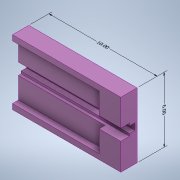
# Autodesk Inventor part: pistonHousing-8-in
Saved by Autodesk Inventor 2020.2 (Build 242310000, 310)
## iProperties
Created: 2020-01-13
Part Number: pistonHousing-8-in
Material: PET Plastic
Document SubType Name: Modeling
Designer: robst
Density: 1.541 g/cm^3
Appearance: Smooth - Purple
Author: robst
Autodesk Inventor part; units mm, degrees
ref_plane "Work Plane1" through (-127, 50.8, 9.525) normal (0, 0, 1) x (1, 0, 0)
sketch "Sketch1" plane through (0, 0, 0) normal (0, 0, 1) x (1, 0, 0)
  line L0 (-127, -76.2) -> (127, -76.2)
  line L1 (127, -76.2) -> (127, 76.2)
  line L2 (127, 76.2) -> (-127, 76.2)
  line L3 (-127, 76.2) -> (-127, -76.2)
  line L4 (-127, -76.2) -> (127, 76.2) construction
  line L5 (127, -76.2) -> (-127, 76.2) construction
  point P0 (0, 0)
  dimension "d0" = 254
  dimension "d1" = 152.4
  constraints: 12 end point, 2 midpoint, 2 parallel, 1 horizontal, 1 perpendicular
  measures "d0" distance of L2.end L1.end
  measures "d1" distance of L1.end L0.end
extrude "Extrusion1" add sketch "Sketch1" along normal mid plane 38.1
sketch "Sketch10" plane through (0, 0, 19.05) normal (0, 0, 1) x (1, 0, 0)
  line L0 (-127, -13.335) -> (127, -13.335)
  line L1 (127, -13.335) -> (127, 13.335)
  line L2 (127, 13.335) -> (-127, 13.335)
  line L3 (-127, 13.335) -> (-127, -13.335)
  line L4 (-127, -13.335) -> (127, 13.335) construction
  line L5 (127, -13.335) -> (-127, 13.335) construction
  line L6 (-127, 76.2) -> (-127, -76.2) projected
  point P0 (0, 0)
  dimension "d71" = 26.67
  constraints: 12 end point, 2 midpoint, 2 parallel, 1 collinear, 1 perpendicular
  measures "d71" distance of L1.end L0.end
extrude "Extrusion7" cut sketch "Sketch10" against normal blind 20.32
ref_plane "Work Plane3" through (0, 0, 0) normal (0, 0, 1) x (1, 0, 0)
ref_plane "Work Plane4" through (0, 0, 19.05) normal (0, 0, 1) x (1, 0, 0)
sketch "Sketch11" plane through (0, 0, -1.27) normal (0, 0, 1) x (1, 0, 0)
  line L0 (-127, -7.62) -> (127, -7.62)
  line L1 (127, -7.62) -> (127, 7.62)
  line L2 (127, 7.62) -> (-127, 7.62)
  line L3 (-127, 7.62) -> (-127, -7.62)
  line L4 (-127, -7.62) -> (127, 7.62) construction
  line L5 (127, -7.62) -> (-127, 7.62) construction
  line L6 (-127, 76.2) -> (-127, 13.335) projected
  point P0 (0, 0)
  dimension "d75" = 15.24
  constraints: 12 end point, 2 midpoint, 2 parallel, 1 collinear, 1 perpendicular
  measures "d75" distance between parallel lines of L2 L0
extrude "Extrusion8" cut sketch "Sketch11" against normal blind 12.7
sketch "Sketch12" plane through (0, 0, 19.05) normal (0, 0, 1) x (1, 0, 0)
  line L0 (-127, 76.2) -> (-127, 13.335) projected
  line L1 (-127, 63.5) -> (76.2, 63.5)
  line L2 (76.2, 63.5) -> (76.2, -63.5)
  line L3 (76.2, -63.5) -> (-127, -63.5)
  line L4 (-127, -63.5) -> (-127, 63.5)
  line L5 (127, 76.2) -> (-127, 76.2) projected
  line L6 (-127, -76.2) -> (127, -76.2) projected
  point P0 (0, 0)
  dimension "d78" = 12.7
  dimension "d79" = 12.7
  dimension "d80" = 203.2
  constraints: 8 end point, 2 parallel, 1 horizontal, 1 perpendicular, 1 point on line
  measures "d78" distance between parallel lines of L5 L1
  measures "d79" distance between parallel lines of L3 L6
  measures "d80" distance between parallel lines of L2 L0
extrude "Extrusion9" cut sketch "Sketch12" against normal blind 13.97
sketch "Sketch3" plane through (0, 0, 19.05) normal (0, 0, 1) x (1, 0, 0)
  line L0 (-76.2, -12.7) -> (76.2, -12.7)
  line L1 (76.2, -12.7) -> (76.2, 12.7)
  line L2 (76.2, 12.7) -> (-76.2, 12.7)
  line L3 (-76.2, 12.7) -> (-76.2, -12.7)
  line L4 (-76.2, -12.7) -> (76.2, 12.7) construction
  line L5 (76.2, -12.7) -> (-76.2, 12.7) construction
  point P0 (0, 0)
  dimension "d7" = 25.4
  dimension "d19" = 152.4
  constraints: 12 end point, 2 midpoint, 2 parallel, 1 horizontal, 1 perpendicular
  measures "d7" distance of L1.end L0.end
  measures "d19" distance of L1.end L2.end
sketch "Sketch8" plane through (0, 0, 19.05) normal (0, 0, 1) x (1, 0, 0)
  line L0 (-76.2, -12.7) -> (-76.2, 12.7) projected
  line L1 (-76.2, 0) -> (38.1, 0)
  line L2 (38.1, 0) -> (38.1, 38.1)
  line L3 (38.1, 38.1) -> (-76.2, 38.1)
  line L4 (-76.2, 38.1) -> (-76.2, 0)
  line L5 (38.1, 0) -> (38.1, -38.1)
  line L6 (38.1, -38.1) -> (-76.2, -38.1)
  line L7 (-76.2, -38.1) -> (-76.2, 0)
  point P0 (0, 0)
  dimension "d51" = 114.3
  dimension "d52" = 38.1
  constraints: 14 end point, 2 parallel, 2 symmetric about line, 1 horizontal, 1 midpoint, 1 perpendicular
  measures "d51" distance of L3.end L2.end
  measures "d52" distance of L2.end L1.end
sketch "Sketch9" plane through (0, 0, 19.05) normal (0, 0, 1) x (1, 0, 0)
  line L0 (-127, 76.2) -> (-127, -76.2) construction
  line L1 (-127, -57.15) -> (127, -57.15) construction
  line L2 (127, 76.2) -> (127, -76.2) construction
  line L3 (-127, -57.15) -> (-127, -44.4609) construction
  point P0 (0, 0)
  point P1 (-127, 76.2)
  point P2 (-76.2, 38.1)
  point P3 (-101.6, -57.15)
  point P4 (-76.2, -57.15)
  point P5 (-50.8, -57.15)
  point P6 (-25.4, -57.15)
  point P7 (0, -57.15)
  point P8 (-101.6, -146.05)
  point P9 (-76.2, -146.05)
  point P10 (-50.8, -146.05)
  point P11 (-25.4, -146.05)
  point P12 (0, -146.05)
  point P13 (-101.6, -234.95)
  point P14 (-76.2, -234.95)
  point P15 (-50.8, -234.95)
  point P16 (-25.4, -234.95)
  point P17 (0, -234.95)
  point P18 (-101.6, -323.85)
  point P19 (-76.2, -323.85)
  point P20 (-50.8, -323.85)
  point P21 (-25.4, -323.85)
  point P22 (0, -323.85)
  point P23 (-127, -76.2)
  dimension "d55" = 25.4
  dimension "d58" = 25.4
  dimension "d61" = 88.9
  constraints: 4 end point, 2 horizontal, 2 point on line, 2 vertical, 21 other
  measures "d58" distance of point (-101.6, -57.15) point (-76.2, -57.15)
  measures "d61" distance of point (-101.6, -57.15) point (-101.6, -146.05)
body "Solid1"
